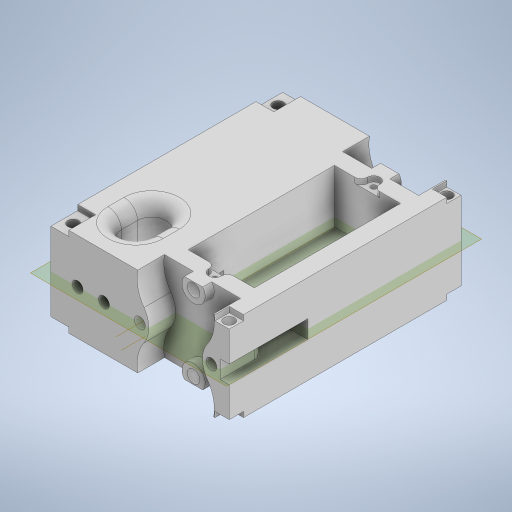
# Autodesk Inventor part: NEW_BODY
Saved by Autodesk Inventor 2024.2 (Build 282272000, 272)
## iProperties
Created: 2024-03-12
Part Number: NEW_BODY
Material: Generic
Document SubType Name: Modeling
Designer: jerem
Density: 1 g/cm^3
Appearance: Default
Author: jerem
## iProperties of the stored document NEW_BODY_3DPrint.ipt
Created: 2024-03-13
Part Number: NEW_BODY_3DPrint
Material: Generic
Document SubType Name: Modeling
Designer: jerem
Density: 1 g/cm^3
Appearance: Default
Author: jerem
Autodesk Inventor part; units mm, degrees
ref_plane "YZ Plane" through (0, 0, 0) normal (1, 0, 0) x (0, 1, 0)
ref_plane "XZ Plane" through (0, 0, 0) normal (0, 1, 0) x (-1, 0, 0)
ref_plane "XY Plane" through (0, 0, 0) normal (0, 0, 1) x (1, 0, 0)
sketch "Sketch1" plane through (0, 0, 0) normal (0, 1, 0) x (-1, 0, 0)
  line L0 (-50, -65) -> (50, -65)
  line L1 (50, -65) -> (50, 65)
  line L2 (50, 65) -> (-50, 65)
  line L3 (-50, 65) -> (-50, -65)
  line L4 (-50, -65) -> (50, 65) construction
  line L5 (50, -65) -> (-50, 65) construction
  point P0 (0, 0)
  dimension "d0" = 130
  dimension "d1" = 100
  constraints: 12 end point, 2 midpoint, 2 parallel, 1 horizontal, 1 perpendicular
  measures "d0" distance of L0.end L1.end
  measures "d1" distance of L1.end L2.end
extrude "Extrusion1" add sketch "Sketch1" along normal blind 50
sketch "Sketch2" plane through (-50, 0, 65) normal (0, 0, 1) x (1, 0, 0)
  line L0 (0, 50) -> (100, 50) projected
  line L1 (100, 50) -> (50, 50)
  line L2 (50, 50) -> (50, 0)
  line L3 (50, 0) -> (100, 0)
  line L4 (100, 0) -> (100, 50)
  constraints: 8 end point, 2 parallel, 1 horizontal, 1 perpendicular
extrude "Extrusion2" cut sketch "Sketch2" against normal blind 15
sketch "Sketch3" plane through (-50, 0, 50) normal (0, 0, 1) x (1, 0, 0)
  circle A0 centre (70, 46.3) radius 3.7
  line L0 (100, 50) -> (100, 0) projected
  line L1 (50, 50) -> (100, 50) projected
  line L2 (50, 0) -> (50, 50) projected
  line L3 (50, 25) -> (100, 25) construction
  circle A1 centre (70, 3.7) radius 3.7
  dimension "d8" = 7.4
  dimension "d95" = 20
  constraints: 2 centre point, 2 end point, 2 midpoint, 1 symmetric about line, 1 tangent, 1 other
  measures "d8" diameter of A0
  measures "d95" distance from line of L2 A0.centre
sketch "Sketch4" plane through (-50, 0, 50) normal (0, 0, 1) x (1, 0, 0)
  circle A0 centre (70, 46.3) radius 3.7 projected
  circle A1 centre (70, 3.7) radius 3.7 projected
  arc A2 (66.7875, 50) -> (73.2125, 50) centre (70, 46.3) ccw
  arc A3 (73.2125, 0) -> (66.7875, 0) centre (70, 3.7) ccw
  line L0 (73.2125, 50) -> (66.7875, 50)
  line L1 (50, 50) -> (100, 50) projected
  line L2 (73.2125, 0) -> (66.7875, 0)
  point P0 (50, 0)
  point P1 (70, 50)
  dimension "d11" = 1.2
  dimension "d12" = 1.2
  dimension "d13" = 6.4249
  dimension "d14" = 6.4249
  constraints: 4 end point, 4 point on circle, 2 centre point, 2 coincident, 1 parallel, 1 point on line, 1 vertical alignment
  measures "d12" radial gap between concentric circles of A1 A3
  measures "d13" distance of L0.start L0.end
  measures "d14" distance of L2.start L2.end
ref_plane "Work Plane1" through (50, 0, 0) normal (0, 0, -1) x (-1, 0, 0)
mirror "Mirror1" about plane through (50, 0, 0) normal (0, 0, -1) of "Extrusion2"
sketch "Sketch5" plane through (0, 0, 0) normal (0, -1, 0) x (1, 0, 0)
  line L0 (-46, -47.5) -> (-4, -47.5)
  line L1 (-4, -47.5) -> (-4, 47.5)
  line L2 (-4, 47.5) -> (-46, 47.5)
  line L3 (-46, 47.5) -> (-46, -47.5)
  line L4 (-46, -47.5) -> (-4, 47.5) construction
  line L5 (-4, -47.5) -> (-46, 47.5) construction
  line L6 (-50, -65) -> (-50, 65) projected
  line L7 (50, 50) -> (50, -50) projected
  line L8 (50, 0) -> (-50, 0) construction
  point P0 (0, 0)
  point P1 (-25, 0)
  dimension "d18" = 4
  dimension "d19" = 42
  dimension "d20" = 95
  constraints: 14 end point, 4 midpoint, 2 parallel, 1 horizontal, 1 perpendicular, 1 point on line
  measures "d18" distance between parallel lines of L6 L3
  measures "d19" distance of L1.end L2.end
  measures "d20" distance of L0.end L1.end
extrude "Extrusion5" cut sketch "Sketch5" against normal blind 27
sketch "Sketch6" plane through (0, 27, 0) normal (0, -1, 0) x (1, 0, 0)
  circle A0 centre (-7.9, -43.6) radius 1.25
  circle A1 centre (-42.1, -43.6) radius 1.25
  circle A2 centre (-42.1, 10.4) radius 1.25
  line L0 (-4, 47.5) -> (-4, -47.5) projected
  line L1 (-46, -47.5) -> (-46, 47.5) projected
  circle A3 centre (-42.1, 10.4) radius 3.9
  circle A4 centre (-42.1, -43.6) radius 3.9
  circle A5 centre (-7.9, -43.6) radius 3.9
  line L2 (-7.9, -43.6) -> (-4, -43.6)
  line L3 (-42.1, -43.6) -> (-46, -43.6)
  line L4 (-4, -47.5) -> (-46, -47.5) projected
  arc A6 (-14.7411, -47.5) -> (-11.7667, -44.1087) centre (-14.7411, -44.5) ccw
  arc A7 (-7.3913, -39.7333) -> (-4, -36.7589) centre (-7, -36.7589) ccw
  arc A8 (-46, -36.7589) -> (-42.6087, -39.7333) centre (-43, -36.7589) ccw
  arc A9 (-38.2333, -44.1087) -> (-35.2589, -47.5) centre (-35.2589, -44.5) ccw
  arc A10 (-42.6087, 6.5333) -> (-46, 3.5589) centre (-43, 3.5589) ccw
  arc A11 (-46, 17.2411) -> (-42.6087, 14.2667) centre (-43, 17.2411) ccw
  point P0 (0, 0)
  point P1 (-42.1, -47.5)
  point P2 (-7.9, -47.5)
  point P3 (-46, 10.4)
  dimension "d23" = 2.5
  dimension "d24" = 2.5
  dimension "d25" = 2.5
  dimension "d26" = 34.2
  dimension "d28" = 54
  dimension "d30" = 34.2
  dimension "d34" = 3
  dimension "d35" = 3
  dimension "d36" = 3
  dimension "d37" = 3
  dimension "d38" = 3
  dimension "d39" = 3
  constraints: 20 point on circle, 17 tangent, 12 centre point, 8 point on line, 4 end point, 3 coincident, 1 collinear
  measures "d23" diameter of A2
  measures "d24" diameter of A0
  measures "d25" diameter of A1
  measures "d26" distance of A1.centre A0.centre
  measures "d28" distance of A2.centre A1.centre
  measures "d30" horizontal distance of A0.centre A2.centre
  measures "d34" radius of A11
  measures "d35" radius of A10
  measures "d36" radius of A8
  measures "d37" radius of A9
  measures "d38" radius of A6
  measures "d39" radius of A7
extrude "Extrusion6" add sketch "Sketch6" along normal blind 8
chamfer "Chamfer1" distance 2 distance2 8 3 edges at (-38.2, 19, 10.4) (-44.9781, 19, 14.9856) (-44.9781, 19, 5.8144) measured on face at (-45.3078, 19, 14.6097) measured on face at (-45.3078, 19, 6.1903) measured on face at (-38.7, 19, 10.4)
chamfer "Chamfer2" distance 2 distance2 8 3 edges at (-10.6577, 19, -40.8423) (-12.4856, 19, -46.4781) (-5.0219, 19, -39.0144) measured on face at (-12.1097, 19, -46.8078) measured on face at (-4.6922, 19, -39.3903) measured on face at (-10.3042, 19, -41.1958)
chamfer "Chamfer3" distance 2 distance2 8 3 edges at (-37.5144, 19, -46.4781) (-39.3423, 19, -40.8423) (-44.9781, 19, -39.0144) measured on face at (-37.8903, 19, -46.8078) measured on face at (-45.3078, 19, -39.3903) measured on face at (-39.6958, 19, -41.1958)
sketch "Sketch7" plane through (0, 50, 0) normal (0, 1, 0) x (1, 0, 0)
  line L0 (-46, 47.5) -> (-46, -47.5) projected
  line L1 (-46, -47.5) -> (-4, -47.5) projected
  line L2 (-4, -47.5) -> (-4, 47.5) projected
  line L3 (-4, 47.5) -> (-46, 47.5) projected
  line L4 (3, 41) -> (40, 41)
  line L5 (40, 41) -> (40, -41)
  line L6 (40, -41) -> (3, -41)
  line L7 (3, -41) -> (3, 41)
  line L8 (3, 41) -> (40, -41) construction
  line L9 (40, 41) -> (3, -41) construction
  line L10 (-46, 0) -> (-4, 0) construction
  line L11 (-4, -47.5) -> (-4, 36.7589) construction
  line L12 (-50, 65) -> (-50, -65) projected
  line L13 (50, -50) -> (50, 50) projected
  point P0 (0, 0)
  point P1 (21.5, 0)
  dimension "d49" = 37
  dimension "d50" = 82
  dimension "d75" = 10
  constraints: 14 end point, 3 midpoint, 2 parallel, 2 perpendicular, 2 point on line, 1 horizontal
  measures "d49" distance of L5.end L6.end
  measures "d50" distance of L4.end L5.end
  measures "d75" distance between parallel lines of L13 L5
extrude "Extrusion7" cut sketch "Sketch7" against normal blind 30 contours L4 L5 L6 L7
sketch "Sketch9" plane through (0, 50, 0) normal (0, 1, 0) x (1, 0, 0)
  circle A0 centre (21.5, -44.5) radius 3.5
  line L0 (40, -41) -> (3, -41) projected
  line L1 (21.5, -44.5) -> (21.5, -41) construction
  line L2 (3, -41) -> (40, -41) construction
  arc A1 (28.5, -41) -> (25, -44.5) centre (28.5, -44.5) ccw
  arc A2 (18, -44.5) -> (14.5, -41) centre (14.5, -44.5) ccw
  line L3 (40, 41) -> (40, -41) construction
  line L4 (40, 0) -> (3, 0) construction
  line L5 (3, -41) -> (3, 41) construction
  circle A3 centre (21.5, 44.5) radius 3.5
  line L6 (21.5, 44.5) -> (21.5, 41) construction
  arc A4 (25, 44.5) -> (28.5, 41) centre (28.5, 44.5) ccw
  arc A5 (14.5, 41) -> (18, 44.5) centre (14.5, 44.5) ccw
  line L7 (28.5, 41) -> (14.5, 41)
  line L8 (3, 41) -> (40, 41) projected
  point P0 (0, 0)
  point P1 (14.5, -41)
  dimension "d60" = 7
  dimension "d62" = 3.5
  dimension "d63" = 3.5
  constraints: 14 point on circle, 10 end point, 9 symmetric about line, 6 centre point, 5 tangent, 4 midpoint, 4 point on line, 2 collinear, 3 other
  measures "d60" diameter of A0
  measures "d62" radius of A1
  measures "d63" radius of A2
extrude "Extrusion9" cut sketch "Sketch9" against normal blind 3
sketch "Sketch10" plane through (0, 0, 0) normal (0, -1, 0) x (1, 0, 0)
  line L0 (-46, -47.5) -> (-46, 47.5) construction
  line L1 (-46, 0) -> (0, 0) construction
  line L2 (-4, -47.5) -> (-46, -47.5) projected
  line L3 (-46, -47.5) -> (-4, -47.5) construction
  circle A0 centre (-25, -52.5) radius 5
  arc A1 (-30, -52.5) -> (-35, -47.5) centre (-35, -52.5) ccw
  arc A2 (-15, -47.5) -> (-20, -52.5) centre (-15, -52.5) ccw
  line L4 (-25, -47.5) -> (-25, -52.5) construction
  line L5 (-14.7411, -47.5) -> (-35.2589, -47.5) construction
  line L6 (-4, 47.5) -> (-46, 47.5)
  line L7 (-46, 47.5) -> (-4, 47.5) construction
  circle A3 centre (-25, 52.5) radius 5
  arc A4 (-35, 47.5) -> (-30, 52.5) centre (-35, 52.5) ccw
  arc A5 (-20, 52.5) -> (-15, 47.5) centre (-15, 52.5) ccw
  line L8 (-25, 47.5) -> (-25, 52.5) construction
  line L9 (-14.7411, 47.5) -> (-35.2589, 47.5) construction
  dimension "d66" = 10
  dimension "d67" = 5
  dimension "d68" = 5
  constraints: 14 end point, 12 point on circle, 12 symmetric about line, 6 centre point, 6 point on line, 5 tangent, 2 horizontal, 2 midpoint, 1 perpendicular, 3 other
  measures "d66" diameter of A0
  measures "d67" radius of A2
  measures "d68" radius of A1
extrude "Extrusion10" cut sketch "Sketch10" against normal blind 3
sketch "Sketch11" plane through (0, 3, 0) normal (0, -1, 0) x (1, 0, 0)
  line L0 (-15, 47.5) -> (-35, 47.5) projected
  arc A0 (-20, 52.5) -> (-15, 47.5) centre (-15, 52.5) ccw projected
  arc A1 (-20, 52.5) -> (-30, 52.5) centre (-25, 52.5) ccw projected
  arc A2 (-35, 47.5) -> (-30, 52.5) centre (-35, 52.5) ccw projected
  line L1 (-35, -47.5) -> (-15, -47.5) projected
  arc A3 (-30, -52.5) -> (-35, -47.5) centre (-35, -52.5) ccw projected
  arc A4 (-30, -52.5) -> (-20, -52.5) centre (-25, -52.5) ccw projected
  arc A5 (-15, -47.5) -> (-20, -52.5) centre (-15, -52.5) ccw projected
  circle A6 centre (-25, -52.5) radius 1.55
  circle A7 centre (-25, 52.5) radius 1.55
  point P0 (0, 0)
  dimension "d71" = 3.1
  dimension "d72" = 3.1
  constraints: 2 centre point, 2 coincident
  measures "d71" diameter of A6
  measures "d72" diameter of A7
extrude "Extrusion11" cut sketch "Sketch11" against normal blind 5 contours A6 | A7
sketch "Sketch13" plane through (0, 20, 0) normal (0, 1, 0) x (1, 0, 0)
  line L0 (3, -41) -> (3, 41) projected
  line L1 (3, -41) -> (13, -41)
  line L2 (13, -41) -> (13, -21)
  line L3 (13, -21) -> (3, -21)
  line L4 (3, -21) -> (3, -41)
  point P0 (0, 0)
  point P1 (3, -21)
  dimension "d76" = 20
  dimension "d77" = 10
  constraints: 8 end point, 2 parallel, 1 horizontal, 1 perpendicular
  measures "d76" distance of L1.end L2.end
  measures "d77" distance of L2.end L3.end
revolve "Revolution1" cut sketch "Sketch13" angle 225 about axis through (3, 20, 41) along (0, 0, 1)
sketch "Sketch15" plane through (0, 47, 0) normal (0, 1, 0) x (1, 0, 0)
  line L0 (14.5, -41) -> (28.5, -41) projected
  arc A0 (18, -44.5) -> (14.5, -41) centre (14.5, -44.5) ccw projected
  arc A1 (18, -44.5) -> (25, -44.5) centre (21.5, -44.5) ccw projected
  arc A2 (28.5, -41) -> (25, -44.5) centre (28.5, -44.5) ccw projected
  arc A3 (25, 44.5) -> (28.5, 41) centre (28.5, 44.5) ccw projected
  arc A4 (25, 44.5) -> (18, 44.5) centre (21.5, 44.5) ccw projected
  arc A5 (14.5, 41) -> (18, 44.5) centre (14.5, 44.5) ccw projected
  line L1 (28.5, 41) -> (14.5, 41) projected
  circle A6 centre (21.5, -44.5) radius 1.55
  circle A7 centre (21.5, 44.5) radius 1.55
  point P0 (0, 0)
  dimension "d79" = 3.1
  dimension "d80" = 3.1
  constraints: 2 centre point, 2 coincident
  measures "d79" diameter of A6
  measures "d80" diameter of A7
extrude "Extrusion12" cut sketch "Sketch15" against normal blind 5 contours A6 | A7
sketch "Sketch16" plane through (40, 50, -41) normal (-1, 0, 0) x (0, 0, 1)
  line L0 (47.5333, -23) -> (49.5162, -31) projected
  line L1 (0, -30) -> (82, -30) projected
  line L2 (82, -30) -> (62, -30)
  line L3 (62, -30) -> (62, -20)
  line L4 (62, -20) -> (82, -20)
  line L5 (82, -20) -> (82, -30)
  point P0 (41, -50)
  dimension "d83" = 20
  dimension "d84" = 10
  constraints: 8 end point, 2 parallel, 1 horizontal, 1 perpendicular
  measures "d83" distance of L3.end L4.end
  measures "d84" distance of L2.end L3.end
extrude "Extrusion13" cut sketch "Sketch16" against normal up to surface (10 mm away)
sketch "Sketch17" plane through (-50, 0, -65) normal (0, 0, -1) x (-1, 0, 0)
  line L0 (0, 0) -> (0, 50) construction
  line L1 (0, 25) -> (-15, 25) construction
  circle A0 centre (-15, 25) radius 3
  line L2 (-15, 25) -> (-29.8, 25) construction
  circle A1 centre (-29.8, 25) radius 3
  point P0 (-50, 0)
  dimension "d87" = 6
  dimension "d88" = 15
  dimension "d145" = 6
  dimension "d146" = 14.8
  constraints: 4 end point, 2 centre point, 2 coincident, 2 horizontal, 1 midpoint
  measures "d87" diameter of A0
  measures "d88" distance of L1.start L1.end
  measures "d145" diameter of A1
  measures "d146" distance of L2.start L2.end
extrude "Extrusion14" cut sketch "Sketch17" against normal blind 10
mirror "Mirror2" about plane through (0, 0, 0) normal (0, 0, 1) of "Extrusion14"
ref_plane "Work Plane3" through (16.7875, 0, -50) normal (0, 0, -1) x (-1, 0, 0)
sketch "Sketch18" plane through (16.7875, 0, -50) normal (0, 0, -1) x (-1, 0, 0)
  circle A0 centre (-3.2125, 46.3) radius 17.5 construction
  circle A1 centre (-3.2125, 3.7) radius 17.5 construction
  line L0 (-33.2125, 50) -> (-33.2125, 0) projected
  line L1 (-33.2125, 0) -> (-33.2125, 50)
  arc A2 (-33.2125, 10) -> (-33.2125, 40) centre (-33.2125, 25) ccw
  line L2 (26.8875, 50) -> (26.8875, 0)
  arc A3 (26.8875, 40) -> (26.8875, 10) centre (26.8875, 25) ccw
  point P0 (16.7875, 0)
  point P1 (-33.2125, 10)
  point P2 (26.8875, 10)
  point P3 (26.8875, 40)
  dimension "d91" = 35
  dimension "d92" = 35
  dimension "d96" = 30
  constraints: 4 centre point, 4 end point, 4 point on circle, 2 point on line, 1 midpoint
  measures "d91" diameter of A0
  measures "d92" diameter of A1
  measures "d96" diameter of A2
extrude "Extrusion15" add sketch "Sketch18" along normal up to surface (15 mm away)
ref_plane "Work Plane4" through (50, 25, -65) normal (0, 0, -1) x (-1, 0, 0)
sketch "Sketch19" plane through (50, 25, -65) normal (0, 0, -1) x (-1, 0, 0)
  arc A0 (0, -15) -> (0, 15) centre (0, 0) ccw construction
  line L0 (0, -15) -> (0, 15) construction
  circle A1 centre (10, 0) radius 3
  circle A2 centre (85, 0) radius 3 construction
  circle A3 centre (50.1, 0) radius 3
  line L1 (15, 0) -> (10, 0)
  arc A4 (50, 11.0901) -> (50, -11.0901) centre (60.1, 0) ccw projected
  line L2 (105.9, -25) -> (-17.65, -25) projected
  point P0 (45.1, 0)
  dimension "d97" = 6
  dimension "d101" = 6
  dimension "d102" = 5
  dimension "d144" = 5
  constraints: 2 centre point, 2 end point, 2 point on circle, 1 coincident, 1 midpoint, 1 parallel, 1 point on line
  measures "d97" diameter of A1
  measures "d101" diameter of A3
  measures "d102" distance of L1.start L1.end
  measures "d144" distance of point (45.1, 0) A3.centre
extrude "Extrusion16" cut sketch "Sketch19" against normal blind 10
sketch "Sketch21" plane through (0, 27, 0) normal (0, -1, 0) x (1, 0, 0)
  line L0 (-33, 42.5) -> (-17, 42.5)
  line L1 (-17, 42.5) -> (-17, 33.5)
  line L2 (-17, 33.5) -> (-33, 33.5)
  line L3 (-33, 33.5) -> (-33, 42.5)
  line L4 (-33, 42.5) -> (-46, 42.5) construction
  line L5 (-46, -47.5) -> (-46, 47.5) construction
  line L6 (-17, 42.5) -> (-4, 42.5) construction
  line L7 (-4, 47.5) -> (-4, -47.5) construction
  line L8 (-15, 47.5) -> (-35, 47.5) construction
  point P0 (0, 0)
  dimension "d108" = 16
  dimension "d109" = 9
  dimension "d110" = 5
  constraints: 12 end point, 3 point on line, 2 horizontal, 2 parallel, 1 collinear, 1 perpendicular
  measures "d108" distance of L0.start L0.end
  measures "d109" distance between parallel lines of L0 L2
  measures "d110" distance between parallel lines of L8 L0
extrude "Extrusion18" cut sketch "Sketch21" against normal blind 13
sketch "Sketch22" plane through (0, 50, 0) normal (0, 1, 0) x (1, 0, 0)
  line L0 (-17, -33.5) -> (-33, -33.5) projected
  line L1 (-17, -42.5) -> (-17, -33.5) projected
  line L2 (-33, -42.5) -> (-17, -42.5) projected
  line L3 (-33, -33.5) -> (-33, -42.5) projected
  arc A0 (-17, -33.5) -> (-33, -33.5) centre (-25, -33.5) ccw
  line L4 (-33, -42.5) -> (-17, -42.5) projected
  arc A1 (-33, -42.5) -> (-17, -42.5) centre (-25, -42.5) ccw
  line L5 (-17, -42.5) -> (-17, -33.5)
  line L6 (-33, -42.5) -> (-33, -33.5)
  point P0 (0, 0)
  constraints: 4 end point, 4 point on circle, 2 centre point, 2 tangent, 1 collinear, 1 vertical
extrude "Extrusion19" cut sketch "Sketch22" against normal blind 20
sketch "Sketch23" plane through (0, 27, 0) normal (0, -1, 0) x (1, 0, 0)
  line L0 (-17, 33.5) -> (-17, 42.5) construction
  line L1 (-17, 38) -> (-14.3, 38) construction
  line L2 (-35.7, 38) -> (-33, 38) construction
  line L3 (-33, 33.5) -> (-33, 42.5) construction
  circle A0 centre (-14.3, 38) radius 1.15
  circle A1 centre (-35.7, 38) radius 1.15
  point P0 (0, 0)
  dimension "d116" = 2.7
  dimension "d117" = 2.7
  dimension "d118" = 2.3
  dimension "d119" = 2.3
  constraints: 4 end point, 2 centre point, 2 coincident, 2 midpoint, 2 perpendicular
  measures "d116" distance of L1.start L1.end
  measures "d117" distance of L2.end L2.start
  measures "d118" diameter of A0
  measures "d119" diameter of A1
extrude "Extrusion20" cut sketch "Sketch23" against normal blind 4
fillet "Fillet4" radius 7.5 4 edges at (-17, 50, 38) (-25, 50, 50.5) (-33, 50, 38) (-25, 50, 25.5)
sketch "Sketch25" plane through (0, 50, 0) normal (0, 1, 0) x (1, 0, 0)
  line L0 (0, 65) -> (-50, 65) projected
  line L1 (-50, 65) -> (-40, 65)
  line L2 (-40, 65) -> (-40, 50)
  line L3 (-40, 50) -> (-50, 50)
  line L4 (-50, 50) -> (-50, 65)
  circle A0 centre (-45, 57.5) radius 3
  line L5 (-50, 65) -> (-50, -65) construction
  line L6 (-50, 0) -> (-20.5898, 0) construction
  point P0 (0, 0)
  point P1 (-30.8869, 65)
  dimension "d129" = 15
  dimension "d130" = 10
  dimension "d131" = 7.5
  dimension "d132" = 6
  dimension "d133" = 5
  constraints: 10 end point, 2 horizontal, 2 parallel, 1 centre point, 1 midpoint, 1 perpendicular
  measures "d129" distance of L1.end L2.end
  measures "d130" distance of L2.end L3.end
  measures "d131" distance from line of L3 A0.centre
  measures "d132" diameter of A0
  measures "d133" distance from line of L2 A0.centre
extrude "Extrusion21" cut sketch "Sketch25" against normal blind 3 contours L2 L3 L4 L0 | A0
extrude "Extrusion22" cut sketch "Sketch25" against normal blind 5 from surface at -3 contours A0
mirror "Mirror4" about plane through (0, 0, 0) normal (0, 0, 1) of "Extrusion21", "Extrusion22"
sketch "Sketch26" plane through (-10.1, 25, -65) normal (0, 0, -1) x (0, -1, 0)
  arc A0 (-11.0901, -10.1) -> (11.0901, -10.1) centre (0, 0) ccw projected
  circle A1 centre (0, -10) radius 3 projected
  circle A2 centre (0, -10) radius 3
  line L0 (0, -10) -> (-11.1803, -10) construction
  line L1 (0, -10) -> (11.1803, -10) construction
  line L2 (-22, 39.9) -> (-22, 29.9) projected
  line L3 (-22, 29.9) -> (-25, 29.9) projected
  line L4 (-25, -10.1) -> (-25, 29.9) projected
  line L5 (-25, -10.1) -> (-11.0901, -10.1) projected
  line L6 (11.0901, -10.1) -> (25, -10.1) projected
  line L7 (25, -10.1) -> (25, 39.9) projected
  line L8 (25, 39.9) -> (-22, 39.9) projected
  point P0 (-10.1, -25)
  constraints: 4 end point, 2 collinear, 2 point on circle, 1 centre point, 1 concentric, 1 horizontal, 1 point on line
extrude "Extrusion23" cut sketch "Sketch26" against normal up to surface (10 mm away) contours A1
ref_plane "Work Plane2" through (0, 25, 0) normal (0, -1, 0) x (1, 0, 0)
mirror "Mirror6" about plane through (0, 25, 0) normal (0, -1, 0) of "Extrusion21", "Extrusion22", "Mirror4"
sketch "Sketch27" plane through (-50, 47, -65) normal (-1, 0, 0) x (0, 0, 1)
  circle A0 centre (65, -22) radius 5
  line L0 (0, -44) -> (0, 0) projected
  line L1 (156, -22) -> (-26, -22) projected
  point P0 (65, -47)
  dimension "d140" = 10
  dimension "d141" = 65
  constraints: 1 centre point, 1 midpoint
  measures "d140" diameter of A0
  measures "d141" distance from line of L0 A0.centre
extrude "Extrusion24" cut sketch "Sketch27" against normal blind 10
mirror "Mirror7" about plane through (0, 0, 0) normal (0, 0, 1) of "Extrusion15"
sketch "Sketch28" plane through (50, 0, -50) normal (0, 0, -1) x (-1, 0, 0)
  circle A0 centre (10, 25) radius 3 projected
  line L0 (10, 25) -> (30, 25) construction
  line L1 (30, 25) -> (30, 46) construction
  circle A1 centre (30, 46) radius 3.5
  circle A2 centre (30, 46) radius 6.5
  line L2 (35.1235, 50) -> (24.8765, 50)
  line L3 (35.5, 50) -> (32, 50) projected
  line L4 (0, 50) -> (50, 50) projected
  point P0 (50, 0)
  dimension "d147" = 20
  dimension "d148" = 21
  dimension "d149" = 7
  dimension "d150" = 3
  constraints: 6 end point, 2 centre point, 2 coincident, 2 point on circle, 1 collinear, 1 horizontal, 1 perpendicular, 1 point on line
  measures "d147" distance of L0.start L0.end
  measures "d148" distance of L0.end L1.end
  measures "d149" diameter of A1
  measures "d150" radial gap between concentric circles of A2 A1
extrude "Extrusion25" add sketch "Sketch28" along normal blind 5 contours A2 L2 picked at (33.2478, 49.4403)
mirror "Mirror8" about plane through (0, 25, 0) normal (0, -1, 0) of "Extrusion25"
mirror "Mirror9" about plane through (0, 0, 0) normal (0, 0, 1) of "Extrusion25", "Mirror8"
mirror "Mirror10" about plane through (0, 0, 0) normal (0, 0, 1) of "Extrusion16"
sketch "Sketch29" plane through (-10.1, 25, -65) normal (0, 0, -1) x (-1, 0, 0)
  arc A0 (-10.1, 11.0901) -> (-10.1, -11.0901) centre (0, 0) ccw projected
  line L0 (29.9, -25) -> (-10.1, -25) projected
  arc A1 (-8.7702, -25) -> (-12.3019, -8.5827) centre (-30.1, -21) ccw
  circle A2 centre (-30.1, -21) radius 3.5 projected
  constraints: 3 point on circle, 1 centre point, 1 concentric, 1 point on line, 1 tangent
sketch "Sketch31" plane through (-50, 0, 50) normal (0, 0, 1) x (1, 0, 0)
  line L0 (100, 50) -> (100, 40) projected
  arc A0 (100, 40) -> (100, 10) centre (100, 25) ccw projected
  line L1 (100, 50) -> (100, 40)
  line L2 (75.1235, 50) -> (100, 50) construction
  arc A1 (87.7115, 33.6019) -> (91.2464, 50) centre (70, 46) ccw
  line L3 (100, 50) -> (91.2464, 50)
  circle A2 centre (70, 46) radius 3.5 projected
  point P0 (50, 0)
  constraints: 4 end point, 3 point on circle, 1 centre point, 1 collinear, 1 concentric, 1 point on line, 1 tangent, 1 vertical
extrude "Extrusion28" add sketch "Sketch31" along normal up to surface (15 mm away) contours L0 A0 A1 L3
mirror "Mirror13" about plane through (0, 25, 0) normal (0, -1, 0) of "Extrusion28"
mirror "Mirror14" about plane through (0, 0, 0) normal (0, 0, 1) of "Extrusion28", "Mirror13"
sketch "Sketch32" plane through (-10.1, 25, -65) normal (0, 0, -1) x (-1, 0, 0)
  circle A0 centre (-30.1, -21) radius 3.5 construction
  line L0 (-30.1, -21) -> (-30.1, 21.2793) construction
  line L1 (-35.1, 22) -> (-28.1, 22) construction
  arc A1 (-8.7702, -25) -> (-12.3019, -8.5827) centre (-30.1, -21) ccw
  arc A2 (-10.1, 11.0901) -> (-10.1, -11.0901) centre (0, 0) ccw projected
  line L2 (-10.1, -25) -> (-10.1, -11.0901)
  line L3 (-10.1, -11.0901) -> (-10.1, -25) construction
  line L4 (-24.9765, -25) -> (-10.1, -25) projected
  line L5 (-10.1, -25) -> (-8.7702, -25)
  point P0 (-51.3464, -25)
  point P1 (-10.1, -12.5762)
  constraints: 8 end point, 3 point on circle, 2 collinear, 1 centre point, 1 concentric, 1 perpendicular, 1 tangent
extrude "Extrusion29" add sketch "Sketch32" against normal up to surface (15 mm away) contours A1 A2 L2
extrude "Extrusion30" cut sketch "Sketch32" against normal up to surface (15 mm away) contours L5 L2 A1
mirror "Mirror15" about plane through (0, 25, 0) normal (0, -1, 0) of "Extrusion29", "Extrusion30"
mirror "Mirror16" about plane through (0, 0, 0) normal (0, 0, 1) of "Extrusion29", "Extrusion30", "Mirror15"
sketch "Sketch33" plane through (50, 0, -65) normal (1, 0, 0) x (0, 0, -1)
  line L0 (-106, 20) -> (-86, 20) projected
  line L1 (-130, 33.6019) -> (-130, 16.3981) projected
  line L2 (-106, 20) -> (-130, 20)
  line L3 (-130, 20) -> (-130, 30)
  line L4 (-130, 30) -> (-106, 30)
  line L5 (-106, 30) -> (-106, 20)
  point P0 (-65, 0)
  dimension "d167" = 10
  constraints: 8 end point, 2 parallel, 1 horizontal, 1 perpendicular, 1 point on line
  measures "d167" distance of L4.end L0.start
extrude "Extrusion31" cut sketch "Sketch33" against normal blind 5
sketch "Sketch34" plane through (0, 0, 0) normal (0, -1, 0) x (1, 0, 0)
  line L0 (50, 65) -> (50, -65) projected
  line L1 (50, -65) -> (42, -65)
  line L2 (42, -65) -> (42, -57)
  line L3 (42, -57) -> (50, -57)
  line L4 (50, -57) -> (50, -65)
  point P0 (0, 0)
  dimension "d170" = 8
  dimension "d171" = 8
  constraints: 8 end point, 2 parallel, 1 horizontal, 1 perpendicular
  measures "d170" distance of L0.end L1.end
  measures "d171" distance of L1.end L2.end
extrude "Extrusion32" cut sketch "Sketch34" against normal blind 3
sketch "Sketch35" plane through (0, 3, 0) normal (0, -1, 0) x (1, 0, 0)
  circle A0 centre (46, -61) radius 3
  line L0 (50, -57) -> (50, -65) projected
  line L1 (50, -65) -> (42, -65) projected
  point P0 (0, 0)
  dimension "d174" = 6
  dimension "d175" = 4
  dimension "d176" = 4
  constraints: 1 centre point
  measures "d174" diameter of A0
  measures "d175" distance from line of L0 A0.centre
  measures "d176" distance from line of L1 A0.centre
extrude "Extrusion33" cut sketch "Sketch35" against normal blind 11
mirror "Mirror17" about plane through (0, 25, 0) normal (0, -1, 0) of "Extrusion32", "Extrusion33"
mirror "Mirror18" about plane through (0, 0, 0) normal (0, 0, 1) of "Extrusion32", "Extrusion33", "Mirror17"
fillet "Fillet5" radius 5 1 edges at (45, 25, 41)
equation "\"d12\" = d11"
equation "\"d24\" = d23"
equation "\"d25\" = d23"
equation "\"d30\" = d26"
equation "\"d35\" = d34"
equation "\"d36\" = d34"
equation "\"d37\" = d34"
equation "\"d38\" = d34"
equation "\"d39\" = d34"
equation "\"d62\" = 0.5 * d60"
equation "\"d63\" = d62"
equation "\"d72\" = d71"
equation "\"d119\" = d118"
equation "\"M4_HOLE_D\" = 3.81"
equation "\"TOL\" = 0.04"
equation "\"M4_INSRT_D\" = 6"
body "Solid1"
